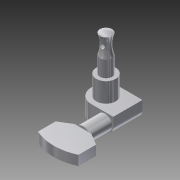
# Autodesk Inventor part: tuning peg
Saved by Autodesk Inventor 2013 (Build 170138000, 138)
## iProperties
Created: 2013-09-11
Part Number: tuning peg
Material: Generic
Document SubType Name: Modeling
Designer: employee
Density: 1 g/cm^3
Author: employee
Autodesk Inventor part; units mm, degrees
ref_plane "YZ Plane" through (0, 0, 0) normal (1, 0, 0) x (0, 1, 0)
ref_plane "XZ Plane" through (0, 0, 0) normal (0, 1, 0) x (-1, 0, 0)
ref_plane "XY Plane" through (0, 0, 0) normal (0, 0, 1) x (1, 0, 0)
sketch "Sketch1" plane through (0, 0, 0) normal (0, 0, 1) x (1, 0, 0)
  line L0 (11.43, 7.62) -> (0, 7.62)
  arc A0 (0, 7.62) -> (0, -7.62) centre (0, 0) ccw
  line L1 (0, -7.62) -> (11.43, -7.62)
  line L2 (11.43, -7.62) -> (11.43, 7.62)
  dimension "d0" = 15.24
  dimension "d2" = 11.43
  constraints: 6 end point, 2 point on circle, 2 tangent, 1 centre point, 1 coincident, 1 horizontal, 1 parallel, 1 perpendicular
  measures "d0" distance between parallel lines of L0 L1
  measures "d2" distance from line of point (0, 0) L2
extrude "Extrusion1" add sketch "Sketch1" along normal blind 8.89
sketch "Sketch2" plane through (0, 0, 8.89) normal (0, 0, 1) x (1, 0, 0)
  arc A0 (0, 7.62) -> (0, -7.62) centre (0, 0) ccw projected
  circle A1 centre (0, 0) radius 5.08
  dimension "d5" = 10.16
  constraints: 1 centre point, 1 coincident
  measures "d5" diameter of A1
extrude "Extrusion2" add sketch "Sketch2" along normal blind 10.16
sketch "Sketch3" plane through (0, 0, 0) normal (0, 1, 0) x (-1, 0, 0)
  line L0 (7.62, 8.89) -> (7.62, 0) projected
  line L1 (7.62, 0) -> (-11.43, 0) projected
  line L2 (-11.43, 0) -> (-11.43, 8.89) projected
  line L3 (-11.43, 8.89) -> (-5.08, 8.89) projected
  line L4 (-5.08, 8.89) -> (-5.08, 19.05) projected
  line L5 (-5.08, 19.05) -> (5.08, 19.05) projected
  line L6 (5.08, 19.05) -> (5.08, 8.89) projected
  line L7 (5.08, 8.89) -> (7.62, 8.89) projected
  line L8 (0, 19.05) -> (0, 38.1)
  arc A0 (3.175, 37.465) -> (0, 38.1) centre (0, 29.845) ccw
  arc A1 (3.175, 37.465) -> (3.175, 27.432) centre (16.8842, 32.4485) ccw
  line L9 (3.175, 27.432) -> (3.175, 19.05)
  line L10 (3.175, 19.05) -> (0, 19.05)
  line L11 (16.8842, 32.4485) -> (2.286, 32.4485)
  point P0 (0, 0)
  dimension "d10" = 3.175
  dimension "d13" = 8.382
  dimension "d14" = 2.286
  dimension "d15" = 19.05
  dimension "d16" = 0.635
  constraints: 8 end point, 5 point on circle, 3 perpendicular, 2 centre point, 2 point on line, 1 midpoint, 1 parallel, 1 vertical alignment
  measures "d10" distance between parallel lines of L9 L8
  measures "d13" distance of L9.start L9.end
  measures "d14" distance from line of L11.end L8
  measures "d15" distance of L8.start L8.end
  measures "d16" vertical distance of L8.end A0.start
revolve "Revolution1" add sketch "Sketch3" angle 360 about axis through (0, 0, 19.05) along (0, 0, 1) contours L5 L8 A0 A1 L9
sketch "Sketch4" plane through (0, 0, 0) normal (0, 1, 0) x (-1, 0, 0)
  line L0 (7.62, 8.89) -> (7.62, 0) projected
  line L1 (7.62, 0) -> (-11.43, 0) projected
  line L2 (-11.43, 0) -> (-11.43, 8.89) projected
  line L3 (-11.43, 8.89) -> (-5.08, 8.89) projected
  line L4 (-5.08, 8.89) -> (-5.08, 19.05) projected
  line L5 (-5.08, 19.05) -> (-3.175, 19.05) projected
  line L6 (-3.175, 19.05) -> (-3.175, 27.432) projected
  arc A0 (-3.175, 27.432) -> (-3.175, 37.465) centre (-16.8842, 32.4485) ccw projected
  arc A1 (3.175, 37.465) -> (0, 38.1) centre (0, 29.845) ccw projected
  arc A2 (0, 38.1) -> (-3.175, 37.465) centre (0, 29.845) ccw projected
  arc A3 (3.175, 37.465) -> (3.175, 27.432) centre (16.8842, 32.4485) ccw projected
  line L7 (3.175, 27.432) -> (3.175, 19.05) projected
  line L8 (3.175, 19.05) -> (5.08, 19.05) projected
  line L9 (5.08, 19.05) -> (5.08, 8.89) projected
  line L10 (5.08, 8.89) -> (7.62, 8.89) projected
  circle A4 centre (0, 32.4485) radius 1.27
  point P0 (0, 0)
  point P1 (2.286, 32.4485)
  dimension "d18" = 2.54
  constraints: 1 centre point, 1 horizontal alignment, 1 point on circle, 1 vertical alignment
  measures "d18" diameter of A4
extrude "Extrusion3" cut sketch "Sketch4" along normal through all both and the other way through all contours A4
sketch "Sketch5" plane through (0, 0, 8.89) normal (0, 0, 1) x (1, 0, 0)
  circle A0 centre (0, 0) radius 5.08 projected
  arc A1 (0, 7.62) -> (0, -7.62) centre (0, 0) ccw projected
  line L0 (-1.7571, 7.4147) -> (-5.8207, 10.24)
  arc A2 (-5.8207, 10.24) -> (-10.24, 5.8207) centre (-7.6332, 7.6332) ccw
  line L1 (-10.24, 5.8207) -> (-7.4147, 1.7571)
  circle A3 centre (-7.6332, 7.6332) radius 1.125
  circle A4 centre (0, 0) radius 10.795
  line L2 (0, 0) -> (-7.6332, 7.6332)
  line L3 (11.43, 7.62) -> (0, 7.62) projected
  dimension "d23" = 2.25
  dimension "d25" = 3.175
  dimension "d26" = 8.001
  dimension "d27" = 5.715
  dimension "d31" = 135
  constraints: 6 end point, 4 point on circle, 2 centre point, 2 coincident, 2 tangent, 1 equal length, 3 other
  measures "d23" diameter of A3
  measures "d25" radius of A2
  measures "d26" distance of L1.end L0.start
  measures "d31" angle of L3 L2
extrude "Extrusion4" add sketch "Sketch5" against normal blind 2.159 contours A1 L1 A4 A3 L2 | L2 A3 A4 L0 A1 | A4 A3 L1 A2 L0
fillet "Fillet1" radius 4.4 1 edges at (11.43, 0, 0)
sketch "Sketch6" plane through (0, -7.62, 8.89) normal (0, -1, 0) x (1, 0, 0)
  arc A0 (7.03, -8.89) -> (11.43, -4.49) centre (7.03, -4.49) ccw projected
  circle A1 centre (7.03, -4.49) radius 3.81
  dimension "d33" = 7.62
  constraints: 1 centre point, 1 coincident
  measures "d33" diameter of A1
extrude "Extrusion5" add sketch "Sketch6" along normal blind 11.43
sketch "Sketch7" plane through (7.03, -19.05, 4.4) normal (0, -1, 0) x (1, 0, 0)
  circle A0 centre (0, 0) radius 3.81 projected
  line L0 (-10.541, 2.54) -> (10.541, 2.54)
  line L1 (10.541, 2.54) -> (10.541, -2.54)
  line L2 (10.541, -2.54) -> (-10.541, -2.54)
  line L3 (-10.541, -2.54) -> (-10.541, 2.54)
  point P0 (-7.03, -4.4)
  point P1 (0, 2.54)
  point P2 (10.541, 0)
  dimension "d37" = 21.082
  dimension "d40" = 5.08
  constraints: 8 end point, 2 midpoint, 2 parallel, 1 horizontal, 1 horizontal alignment, 1 perpendicular, 1 vertical alignment
  measures "d37" distance of L1.end L2.end
  measures "d40" distance between parallel lines of L0 L2
extrude "Extrusion6" add sketch "Sketch7" along normal blind 15.24 contours A0 L2 L0 | A0 L0 L1 L2 | A0 L2 L3 L0
sketch "Sketch8" plane through (-3.511, -19.05, 6.94) normal (0, 0, 1) x (1, 0, 0)
  line L0 (0, 0) -> (7.7012, 0) projected
  line L1 (0, 0) -> (0, -15.24) projected
  line L2 (21.082, -15.24) -> (0, -15.24) projected
  line L3 (21.082, 0) -> (21.082, -15.24) projected
  line L4 (13.3808, 0) -> (21.082, 0) projected
  line L5 (7.7012, 0) -> (13.3808, 0) projected
  line L6 (6.1817, 0) -> (0, -3.7039)
  line L7 (14.9003, 0) -> (21.082, -3.7039)
  arc A0 (0, -12.9438) -> (21.082, -12.9438) centre (10.541, 10.1034) ccw
  point P0 (3.511, 19.05)
  constraints: 6 point on line, 4 end point, 2 horizontal alignment, 2 point on circle, 1 centre point, 1 equal length, 1 tangent
extrude "Extrusion7" cut sketch "Sketch8" against normal through all contours L0 L6 L1 | A0 L2 L1 | A0 L3 L2 | L4 L3 L7
body "Solid1"
